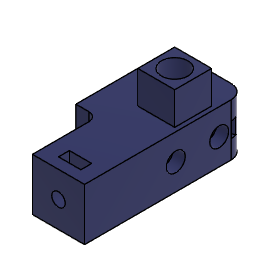
Junta_esquina_laser V4 - Contensor de correa v4 (Autodesk Fusion 360 design; units mm, degrees)
Autodesk Fusion 360 part; units mm, degrees
sketch "Sketch1" plane through (0, 0, 0) normal (0, 0, 1) x (1, 0, 0)
  line L0 (6.2109, 74.5616) -> (40.2109, 74.5616)
  line L1 (40.2109, 74.5616) -> (40.2109, 0.5616)
  line L2 (40.2109, 0.5616) -> (16.2109, 0.5616)
  line L3 (16.2109, 0.5616) -> (16.2109, 30.5616)
  line L4 (16.2109, 30.5616) -> (6.2109, 30.5616)
  line L5 (6.2109, 30.5616) -> (6.2109, 74.5616)
  dimension "d2" = 44
  dimension "d3" = 74
  dimension "d4" = 24
  dimension "d62" = 10
  constraint horizontal L0
  constraint perpendicular L0 L1
  constraint perpendicular L1 L2
  constraint perpendicular L2 L3
  constraint perpendicular L3 L4
  constraint perpendicular L0 L5
  measures "d2" distance of L0.start L4.end
  measures "d3" distance of L0.end L1.end
  measures "d4" distance of L1.end L2.end
  measures "d62" distance of L3.end L4.end
extrude "Extrude1" add sketch "Sketch1" along normal blind 24
sketch "Sketch2" plane through (6.2109, 0, 0) normal (-1, 0, 0) x (0, -1, 0)
  line L0 (-74.5616, 0) -> (-30.5616, 0)
  line L1 (-30.5616, 0) -> (-30.5616, 24)
  line L2 (-30.5616, 24) -> (-74.5616, 24)
  line L3 (-74.5616, 24) -> (-74.5616, 0)
  line L4 (-72.6616, 22.1) -> (-32.4616, 22.1)
  line L5 (-32.4616, 22.1) -> (-32.4616, 1.9)
  line L6 (-32.4616, 1.9) -> (-72.6616, 1.9)
  line L7 (-72.6616, 1.9) -> (-72.6616, 22.1)
  dimension "d7" = 20.2
  dimension "d8" = 40.2
  dimension "d9" = 1.9
  dimension "d10" = 1.9
  constraint horizontal L4
  constraint vertical L5
  constraint horizontal L6
  constraint vertical L7
  measures "d7" distance of L4.start L6.end
  measures "d8" distance of L4.start L4.end
  measures "d9" horizontal distance of L0.start L6.end
  measures "d10" vertical distance of L0.start L6.end
extrude "Extrude2" cut sketch "Sketch2" against normal blind 10 contours L4 L5 L6 L7
sketch "Sketch4" plane through (40.2109, 0, 0) normal (1, 0, 0) x (0, 1, 0)
  line L0 (0.5616, 0) -> (74.5616, 0)
  line L1 (74.5616, 0) -> (74.5616, 24)
  line L2 (74.5616, 24) -> (0.5616, 24)
  line L3 (0.5616, 24) -> (0.5616, 0)
  line L4 (72.5616, 22) -> (32.5616, 22) construction
  line L5 (32.5616, 22) -> (32.5616, 2) construction
  line L6 (32.5616, 2) -> (72.5616, 2) construction
  line L7 (72.5616, 2) -> (72.5616, 22) construction
  circle A0 centre (42.5616, 12) radius 2.6
  circle A1 centre (62.5616, 12) radius 2.6
  line L8 (42.5616, 12) -> (62.5616, 12) construction
  circle A2 centre (42.5616, 12) radius 4.35
  circle A3 centre (62.5616, 12) radius 4.35
  dimension "d18" = 40
  dimension "d19" = 20
  dimension "d20" = 2
  dimension "d21" = 2
  dimension "d22" = 5.2
  dimension "d23" = 10
  dimension "d24" = 10
  dimension "d25" = 20
  dimension "d26" = 8.7
  dimension "d27" = 8.7
  constraint horizontal L4
  constraint vertical L5
  constraint horizontal L6
  constraint vertical L7
  constraint coincident A0.centre L8.start
  constraint coincident A1.centre L8.end
  constraint horizontal L8
  constraint equal A0 A1
  constraint concentric A0 A2
  constraint concentric A1 A3
  measures "d18" distance of L4.start L4.end
  measures "d19" distance of L4.start L6.end
  measures "d20" horizontal distance of L1.end L4.start
  measures "d21" vertical distance of L1.end L4.start
  measures "d22" diameter of A0
  measures "d23" vertical distance of L4.start A1.centre
  measures "d24" horizontal distance of L6.end A1.centre
  measures "d25" distance of A0.centre A1.centre
  measures "d26" diameter of A2
  measures "d27" diameter of A3
extrude "Extrude4" cut sketch "Sketch4" against normal blind 40 contours A0 | A1
extrude "Extrude5" cut sketch "Sketch4" against normal blind 5.5 contours A2 | A3
sketch "Sketch5" plane through (0, 0, 24) normal (0, 0, 1) x (-1, 0, 0)
  line L0 (-6.2109, -30.5616) -> (-16.2109, -30.5616)
  line L1 (-16.2109, -30.5616) -> (-16.2109, -0.5616)
  line L2 (-16.2109, -0.5616) -> (-40.2109, -0.5616)
  line L3 (-40.2109, -0.5616) -> (-40.2109, -74.5616)
  line L4 (-40.2109, -74.5616) -> (-6.2109, -74.5616)
  line L5 (-6.2109, -74.5616) -> (-6.2109, -30.5616)
  circle A0 centre (-29.7109, -52.5616) radius 6.1
  line L6 (-21.2109, -61.0616) -> (-38.2109, -61.0616)
  line L7 (-38.2109, -61.0616) -> (-38.2109, -44.0616)
  line L8 (-38.2109, -44.0616) -> (-21.2109, -44.0616)
  line L9 (-21.2109, -44.0616) -> (-21.2109, -61.0616)
  line L10 (-21.2109, -61.0616) -> (-38.2109, -44.0616) construction
  line L11 (-21.2109, -44.0616) -> (-38.2109, -61.0616) construction
  dimension "d32" = 12.2
  dimension "d33" = 22
  dimension "d35" = 17
  dimension "d36" = 2
  constraint horizontal L6
  constraint vertical L7
  constraint horizontal L8
  constraint vertical L9
  constraint equal L6 L9
  constraint midpoint A0.centre L10
  measures "d32" diameter of A0
  measures "d33" vertical distance of L3.end A0.centre
  measures "d35" distance of L6.start L8.end
  measures "d36" horizontal distance of L3.end L6.end
extrude "Extrude6" cut sketch "Sketch5" against normal blind 32 contours A0
extrude "Extrude7" add sketch "Sketch5" along normal blind 15 contours L6 L7 L8 L9
sketch "Sketch6" plane through (0, 0.5616, 0) normal (0, -1, 0) x (1, 0, 0)
  line L0 (16.2109, 0) -> (40.2109, 0)
  line L1 (40.2109, 0) -> (40.2109, 24)
  line L2 (40.2109, 24) -> (16.2109, 24)
  line L3 (16.2109, 24) -> (16.2109, 0)
  circle A0 centre (28.2109, 12) radius 3.1
  line L4 (16.2109, 24) -> (40.2109, 0) construction
  line L5 (40.2109, 24) -> (16.2109, 0) construction
  dimension "d42" = 6.2
  constraint coincident L2.end L3.start
  constraint coincident L0.end L1.start
  constraint coincident L1.end L2.start
  constraint coincident L0.start L3.end
  constraint midpoint A0.centre L4
  measures "d42" diameter of A0
extrude "Extrude8" cut sketch "Sketch6" against normal blind 26 contours A0
sketch "Sketch7" plane through (0, 0, 24) normal (0, 0, 1) x (-1, 0, 0)
  line L0 (-40.2109, -74.5616) -> (-6.2109, -74.5616)
  line L1 (-6.2109, -74.5616) -> (-6.2109, -30.5616)
  line L2 (-16.2109, -30.5616) -> (-16.2109, -0.5616)
  line L3 (-16.2109, -0.5616) -> (-40.2109, -0.5616)
  line L4 (-40.2109, -0.5616) -> (-40.2109, -74.5616)
  line L5 (-21.2109, -44.0616) -> (-21.2109, -61.0616)
  line L6 (-21.2109, -61.0616) -> (-38.2109, -61.0616)
  line L7 (-38.2109, -61.0616) -> (-38.2109, -44.0616)
  line L8 (-38.2109, -44.0616) -> (-21.2109, -44.0616)
  line L9 (-23.2109, -10.5616) -> (-33.5109, -10.5616)
  line L10 (-33.5109, -10.5616) -> (-33.5109, -5.5616)
  line L11 (-33.5109, -5.5616) -> (-23.2109, -5.5616)
  line L12 (-23.2109, -5.5616) -> (-23.2109, -10.5616)
  line L13 (-6.2109, -30.5616) -> (-16.2109, -30.5616)
  dimension "d45" = 5
  dimension "d46" = 10.3
  dimension "d47" = 7
  dimension "d48" = 5
  constraint horizontal L9
  constraint vertical L10
  constraint horizontal L11
  constraint vertical L12
  measures "d45" distance of L9.start L11.end
  measures "d46" distance of L9.start L9.end
  measures "d47" horizontal distance of L2.end L11.end
  measures "d48" vertical distance of L2.end L11.end
extrude "Extrude9" cut sketch "Sketch7" against normal blind 18 contours L9 L10 L11 L12
sketch "Sketch8" plane through (0, 74.5616, 0) normal (0, 1, 0) x (-1, 0, 0)
  line L0 (-40.2109, 0) -> (-6.2109, 0)
  line L1 (-6.2109, 0) -> (-6.2109, 24)
  line L2 (-6.2109, 24) -> (-40.2109, 24)
  circle A0 centre (-10, 11.5) radius 2.05
  line L3 (-40.2109, 24) -> (-40.2109, 0)
  dimension "d52" = 4.1
  dimension "d53" = 12.5
  dimension "d54" = 10
  measures "d52" diameter of A0
  measures "d53" vertical distance of L1.end A0.centre
  measures "d54" horizontal distance of origin A0.centre
extrude "Extrude10" cut sketch "Sketch8" against normal blind 55 contours A0
sketch "Sketch9" plane through (16.2109, 0, 0) normal (-1, 0, 0) x (0, -1, 0)
  circle A0 centre (-62.5616, 12) radius 2.6
  circle A1 centre (-42.5616, 12) radius 2.6
  line L0 (-72.6616, 1.9) -> (-32.4616, 1.9)
  line L1 (-32.4616, 1.9) -> (-32.4616, 22.1)
  line L2 (-32.4616, 22.1) -> (-72.6616, 22.1)
  line L3 (-72.6616, 22.1) -> (-72.6616, 1.9)
  line L4 (-70.1616, 15.5) -> (-68.1616, 15.5)
  line L5 (-68.1616, 15.5) -> (-68.1616, 8.5)
  line L6 (-68.1616, 8.5) -> (-70.1616, 8.5)
  line L7 (-70.1616, 8.5) -> (-70.1616, 15.5)
  dimension "d57" = 7
  dimension "d58" = 2
  dimension "d59" = 6.6
  dimension "d63" = 2.5
  constraint horizontal L4
  constraint vertical L5
  constraint horizontal L6
  constraint vertical L7
  measures "d57" distance of L4.start L6.end
  measures "d58" distance of L4.start L4.end
  measures "d59" vertical distance of L0.start L6.end
  measures "d63" horizontal distance of L6.end L0.start
extrude "Extrude11" cut sketch "Sketch9" against normal blind 46 contours L4 L5 L6 L7
fillet "Fillet2" radius 1.75 4 edges at (16.2109, 70.1616, 12) (16.2109, 69.1616, 15.5) (16.2109, 68.1616, 12) (16.2109, 69.1616, 8.5)
fillet "Fillet3" radius 2 1 edges at (40.2109, 70.1616, 12)
fillet "Fillet4" radius 4 1 edges at (16.2109, 30.5616, 12)
fillet "Fillet5" radius 6.5 1 edges at (40.2109, 74.5616, 12)
sketch "Sketch3" plane through (0, 74.5616, 0) normal (0, 1, 0) x (-1, 0, 0)
  line L0 (-40.2109, 0) -> (-0.2109, 0)
  line L1 (-0.2109, 0) -> (-0.2109, 24)
  line L2 (-0.2109, 24) -> (-40.2109, 24)
  line L3 (-40.2109, 24) -> (-40.2109, 0)
  circle A0 centre (-4, 12) radius 2.1
  dimension "d13" = 4.2
  dimension "d14" = 12
  dimension "d15" = 4
  measures "d13" diameter of A0
  measures "d14" vertical distance of origin A0.centre
  measures "d15" horizontal distance of origin A0.centre
extrude "Extrude3" [suppressed]
named bodies: "Junta_esquina"
